N35 8x4mm_v2 (Autodesk Fusion 360 design; units mm, degrees)
Autodesk Fusion 360 part; units mm, degrees
sketch "Skizze1" plane through (0, 0, 0) normal (0, 0, 1) x (1, 0, 0)
  circle A0 centre (0, 0) radius 4
  dimension "d1" = 8
  constraint coincident A0.centre origin
  measures "d1" diameter of A0
extrude "Extrusion1" add sketch "Skizze1" along normal blind 4
